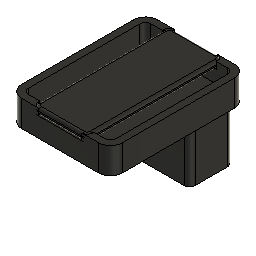
IMUmount (Autodesk Fusion 360 design; units mm, degrees)
Autodesk Fusion 360 part; units mm, degrees
sketch "Sketch1" plane through (0, 0, -6.0198) normal (0, 0, 1) x (-1, 0, 0)
  line L0 (-4.0409, -57.15) -> (2.9359, -57.15)
  line L1 (2.9359, -57.15) -> (3.9347, -56.1512)
  line L2 (3.9347, -56.1512) -> (3.9347, 6.35)
  line L3 (3.9347, 6.35) -> (-16.6393, 6.35)
  line L4 (-16.6393, 6.35) -> (-16.6393, -56.1512)
  line L5 (-16.6393, -56.1512) -> (-15.6405, -57.15)
  line L6 (-15.6405, -57.15) -> (-8.6637, -57.15)
  line L7 (-8.6637, -57.15) -> (-8.6637, -55.3466)
  arc A0 (-8.1557, -54.8386) -> (-8.6637, -55.3466) centre (-8.1557, -55.3466) ccw
  line L8 (-8.1557, -54.8386) -> (-4.5489, -54.8386)
  arc A1 (-4.0409, -55.3466) -> (-4.5489, -54.8386) centre (-4.5489, -55.3466) ccw
  line L9 (-4.0409, -55.3466) -> (-4.0409, -57.15)
  arc A2 (-8.1557, -42.1386) -> (-8.6637, -42.6466) centre (-8.1557, -42.6466) ccw
  line L10 (-8.1557, -42.1386) -> (-4.5489, -42.1386)
  arc A3 (-4.0409, -42.6466) -> (-4.5489, -42.1386) centre (-4.5489, -42.6466) ccw
  line L11 (-4.0409, -42.6466) -> (-4.0409, -46.2534)
  arc A4 (-4.5489, -46.7614) -> (-4.0409, -46.2534) centre (-4.5489, -46.2534) ccw
  line L12 (-4.5489, -46.7614) -> (-8.1557, -46.7614)
  arc A5 (-8.6637, -46.2534) -> (-8.1557, -46.7614) centre (-8.1557, -46.2534) ccw
  line L13 (-8.6637, -46.2534) -> (-8.6637, -42.6466)
  arc A6 (-8.1557, -29.4386) -> (-8.6637, -29.9466) centre (-8.1557, -29.9466) ccw
  line L14 (-8.1557, -29.4386) -> (-4.5489, -29.4386)
  arc A7 (-4.0409, -29.9466) -> (-4.5489, -29.4386) centre (-4.5489, -29.9466) ccw
  line L15 (-4.0409, -29.9466) -> (-4.0409, -33.5534)
  arc A8 (-4.5489, -34.0614) -> (-4.0409, -33.5534) centre (-4.5489, -33.5534) ccw
  line L16 (-4.5489, -34.0614) -> (-8.1557, -34.0614)
  arc A9 (-8.6637, -33.5534) -> (-8.1557, -34.0614) centre (-8.1557, -33.5534) ccw
  line L17 (-8.6637, -33.5534) -> (-8.6637, -29.9466)
  arc A10 (1.8011, -53.1114) -> (2.3091, -52.6034) centre (1.8011, -52.6034) ccw
  line L18 (1.8011, -53.1114) -> (-1.8057, -53.1114)
  arc A11 (-2.3137, -52.6034) -> (-1.8057, -53.1114) centre (-1.8057, -52.6034) ccw
  line L19 (-2.3137, -52.6034) -> (-2.3137, -48.9966)
  arc A12 (-1.8057, -48.4886) -> (-2.3137, -48.9966) centre (-1.8057, -48.9966) ccw
  line L20 (-1.8057, -48.4886) -> (1.8011, -48.4886)
  arc A13 (2.3091, -48.9966) -> (1.8011, -48.4886) centre (1.8011, -48.9966) ccw
  line L21 (2.3091, -48.9966) -> (2.3091, -52.6034)
  arc A14 (1.8011, -40.4114) -> (2.3091, -39.9034) centre (1.8011, -39.9034) ccw
  line L22 (1.8011, -40.4114) -> (-1.8057, -40.4114)
  arc A15 (-2.3137, -39.9034) -> (-1.8057, -40.4114) centre (-1.8057, -39.9034) ccw
  line L23 (-2.3137, -39.9034) -> (-2.3137, -36.2966)
  arc A16 (-1.8057, -35.7886) -> (-2.3137, -36.2966) centre (-1.8057, -36.2966) ccw
  line L24 (-1.8057, -35.7886) -> (1.8011, -35.7886)
  arc A17 (2.3091, -36.2966) -> (1.8011, -35.7886) centre (1.8011, -36.2966) ccw
  line L25 (2.3091, -36.2966) -> (2.3091, -39.9034)
  arc A18 (1.8011, -27.7114) -> (2.3091, -27.2034) centre (1.8011, -27.2034) ccw
  line L26 (1.8011, -27.7114) -> (-1.8057, -27.7114)
  arc A19 (-2.3137, -27.2034) -> (-1.8057, -27.7114) centre (-1.8057, -27.2034) ccw
  line L27 (-2.3137, -27.2034) -> (-2.3137, -23.5966)
  arc A20 (-1.8057, -23.0886) -> (-2.3137, -23.5966) centre (-1.8057, -23.5966) ccw
  line L28 (-1.8057, -23.0886) -> (1.8011, -23.0886)
  arc A21 (2.3091, -23.5966) -> (1.8011, -23.0886) centre (1.8011, -23.5966) ccw
  line L29 (2.3091, -23.5966) -> (2.3091, -27.2034)
  arc A22 (1.8011, -15.0114) -> (2.3091, -14.5034) centre (1.8011, -14.5034) ccw
  line L30 (1.8011, -15.0114) -> (-1.8057, -15.0114)
  arc A23 (-2.3137, -14.5034) -> (-1.8057, -15.0114) centre (-1.8057, -14.5034) ccw
  line L31 (-2.3137, -14.5034) -> (-2.3137, -10.8966)
  arc A24 (-1.8057, -10.3886) -> (-2.3137, -10.8966) centre (-1.8057, -10.8966) ccw
  line L32 (-1.8057, -10.3886) -> (1.8011, -10.3886)
  arc A25 (2.3091, -10.8966) -> (1.8011, -10.3886) centre (1.8011, -10.8966) ccw
  line L33 (2.3091, -10.8966) -> (2.3091, -14.5034)
  arc A26 (1.8011, -2.3114) -> (2.3091, -1.8034) centre (1.8011, -1.8034) ccw
  line L34 (1.8011, -2.3114) -> (-1.8057, -2.3114)
  arc A27 (-2.3137, -1.8034) -> (-1.8057, -2.3114) centre (-1.8057, -1.8034) ccw
  line L35 (-2.3137, -1.8034) -> (-2.3137, 1.8034)
  arc A28 (-1.8057, 2.3114) -> (-2.3137, 1.8034) centre (-1.8057, 1.8034) ccw
  line L36 (-1.8057, 2.3114) -> (1.8011, 2.3114)
  arc A29 (2.3091, 1.8034) -> (1.8011, 2.3114) centre (1.8011, 1.8034) ccw
  line L37 (2.3091, 1.8034) -> (2.3091, -1.8034)
  arc A30 (-10.8989, -53.1114) -> (-10.3909, -52.6034) centre (-10.8989, -52.6034) ccw
  line L38 (-10.8989, -53.1114) -> (-14.5057, -53.1114)
  arc A31 (-15.0137, -52.6034) -> (-14.5057, -53.1114) centre (-14.5057, -52.6034) ccw
  line L39 (-15.0137, -52.6034) -> (-15.0137, -48.9966)
  arc A32 (-14.5057, -48.4886) -> (-15.0137, -48.9966) centre (-14.5057, -48.9966) ccw
  line L40 (-14.5057, -48.4886) -> (-10.8989, -48.4886)
  arc A33 (-10.3909, -48.9966) -> (-10.8989, -48.4886) centre (-10.8989, -48.9966) ccw
  line L41 (-10.3909, -48.9966) -> (-10.3909, -52.6034)
  arc A34 (-10.8989, -40.4114) -> (-10.3909, -39.9034) centre (-10.8989, -39.9034) ccw
  line L42 (-10.8989, -40.4114) -> (-14.5057, -40.4114)
  arc A35 (-15.0137, -39.9034) -> (-14.5057, -40.4114) centre (-14.5057, -39.9034) ccw
  line L43 (-15.0137, -39.9034) -> (-15.0137, -36.2966)
  arc A36 (-14.5057, -35.7886) -> (-15.0137, -36.2966) centre (-14.5057, -36.2966) ccw
  line L44 (-14.5057, -35.7886) -> (-10.8989, -35.7886)
  arc A37 (-10.3909, -36.2966) -> (-10.8989, -35.7886) centre (-10.8989, -36.2966) ccw
  line L45 (-10.3909, -36.2966) -> (-10.3909, -39.9034)
  arc A38 (-10.8989, -27.7114) -> (-10.3909, -27.2034) centre (-10.8989, -27.2034) ccw
  line L46 (-10.8989, -27.7114) -> (-14.5057, -27.7114)
  arc A39 (-15.0137, -27.2034) -> (-14.5057, -27.7114) centre (-14.5057, -27.2034) ccw
  line L47 (-15.0137, -27.2034) -> (-15.0137, -23.5966)
  arc A40 (-14.5057, -23.0886) -> (-15.0137, -23.5966) centre (-14.5057, -23.5966) ccw
  line L48 (-14.5057, -23.0886) -> (-10.8989, -23.0886)
  arc A41 (-10.3909, -23.5966) -> (-10.8989, -23.0886) centre (-10.8989, -23.5966) ccw
  line L49 (-10.3909, -23.5966) -> (-10.3909, -27.2034)
  arc A42 (-10.8989, -15.0114) -> (-10.3909, -14.5034) centre (-10.8989, -14.5034) ccw
  line L50 (-10.8989, -15.0114) -> (-14.5057, -15.0114)
  arc A43 (-15.0137, -14.5034) -> (-14.5057, -15.0114) centre (-14.5057, -14.5034) ccw
  line L51 (-15.0137, -14.5034) -> (-15.0137, -10.8966)
  arc A44 (-14.5057, -10.3886) -> (-15.0137, -10.8966) centre (-14.5057, -10.8966) ccw
  line L52 (-14.5057, -10.3886) -> (-10.8989, -10.3886)
  arc A45 (-10.3909, -10.8966) -> (-10.8989, -10.3886) centre (-10.8989, -10.8966) ccw
  line L53 (-10.3909, -10.8966) -> (-10.3909, -14.5034)
  arc A46 (-10.8989, -2.3114) -> (-10.3909, -1.8034) centre (-10.8989, -1.8034) ccw
  line L54 (-10.8989, -2.3114) -> (-14.5057, -2.3114)
  arc A47 (-15.0137, -1.8034) -> (-14.5057, -2.3114) centre (-14.5057, -1.8034) ccw
  line L55 (-15.0137, -1.8034) -> (-15.0137, 1.8034)
  arc A48 (-14.5057, 2.3114) -> (-15.0137, 1.8034) centre (-14.5057, 1.8034) ccw
  line L56 (-14.5057, 2.3114) -> (-10.8989, 2.3114)
  arc A49 (-10.3909, 1.8034) -> (-10.8989, 2.3114) centre (-10.8989, 1.8034) ccw
  line L57 (-10.3909, 1.8034) -> (-10.3909, -1.8034)
  arc A50 (-8.6637, -8.1534) -> (-8.1557, -8.6614) centre (-8.1557, -8.1534) ccw
  line L58 (-8.6637, -8.1534) -> (-8.6637, -4.5466)
  arc A51 (-8.1557, -4.0386) -> (-8.6637, -4.5466) centre (-8.1557, -4.5466) ccw
  line L59 (-8.1557, -4.0386) -> (-4.5489, -4.0386)
  arc A52 (-4.0409, -4.5466) -> (-4.5489, -4.0386) centre (-4.5489, -4.5466) ccw
  line L60 (-4.0409, -4.5466) -> (-4.0409, -8.1534)
  arc A53 (-4.5489, -8.6614) -> (-4.0409, -8.1534) centre (-4.5489, -8.1534) ccw
  line L61 (-4.5489, -8.6614) -> (-8.1557, -8.6614)
  arc A54 (-8.1557, -16.7386) -> (-8.6637, -17.2466) centre (-8.1557, -17.2466) ccw
  line L62 (-8.1557, -16.7386) -> (-4.5489, -16.7386)
  arc A55 (-4.0409, -17.2466) -> (-4.5489, -16.7386) centre (-4.5489, -17.2466) ccw
  line L63 (-4.0409, -17.2466) -> (-4.0409, -20.8534)
  arc A56 (-4.5489, -21.3614) -> (-4.0409, -20.8534) centre (-4.5489, -20.8534) ccw
  line L64 (-4.5489, -21.3614) -> (-8.1557, -21.3614)
  arc A57 (-8.6637, -20.8534) -> (-8.1557, -21.3614) centre (-8.1557, -20.8534) ccw
  line L65 (-8.6637, -20.8534) -> (-8.6637, -17.2466)
  line L66 (2.6647, -56.1512) -> (-15.3693, -56.1512)
  line L67 (-16.6393, -54.8812) -> (-16.6393, -47.2612)
  line L68 (-15.3693, -45.9912) -> (2.6647, -45.9912)
  line L69 (3.9347, -47.2612) -> (3.9347, -54.8812)
  arc A58 (2.6647, -56.1512) -> (3.9347, -54.8812) centre (2.6647, -54.8812) ccw
  arc A59 (3.9347, -47.2612) -> (2.6647, -45.9912) centre (2.6647, -47.2612) ccw
  arc A60 (-15.3693, -45.9912) -> (-16.6393, -47.2612) centre (-15.3693, -47.2612) ccw
  arc A61 (-16.6393, -54.8812) -> (-15.3693, -56.1512) centre (-15.3693, -54.8812) ccw
  point P0 (-16.6393, -56.1512)
  point P1 (-16.6393, -45.9912)
  dimension "d1" = 10.16
  dimension "d2" = 1.27
  constraint coincident P0 L4.end
  constraint coincident L4 P1
  constraint perpendicular L2 L68
  constraint tangent L66 A58
  constraint tangent L69 A58
  constraint tangent L68 A59
  constraint tangent L69 A59
  constraint equal A58 A59
  constraint coincident P1 L67
  constraint coincident P1 L68
  constraint tangent L67 A60
  constraint tangent L68 A60
  constraint equal A58 A60
  constraint coincident P0 L66
  constraint coincident P0 L67
  constraint tangent L66 A61
  constraint tangent L67 A61
  constraint equal A58 A61
  measures "d1" distance of P0 P1
  measures "d2" radius of A58
extrude "Extrude1" add sketch "Sketch1" along normal blind 12.7 contours L7 A0 L8 A1 L9 L66 | L2 L4 L7 A0 L8 A1 L9 L11 A4 L12 A5 L13 L66 L67 L68 L69 A58 A59 A60 A61 | L11 A4 L12 A5 L13 L68 | A10 L18 A11 L19 A12 L20 A13 L21 | A30 L38 A31 L39 A32 L40 A33 L41 makes body 1
sketch "Sketch2" plane through (0, 0, 6.6802) normal (0, 0, 1) x (-1, 0, 0)
  arc A0 (-15.3693, -45.9912) -> (-16.6393, -47.2612) centre (-15.3693, -47.2612) ccw
  line L0 (-16.6393, -47.2612) -> (-16.6393, -54.8812)
  arc A1 (-16.6393, -54.8812) -> (-15.3693, -56.1512) centre (-15.3693, -54.8812) ccw
  line L1 (-15.3693, -56.1512) -> (2.6647, -56.1512)
  arc A2 (2.6647, -56.1512) -> (3.9347, -54.8812) centre (2.6647, -54.8812) ccw
  line L2 (3.9347, -54.8812) -> (3.9347, -47.2612)
  arc A3 (3.9347, -47.2612) -> (2.6647, -45.9912) centre (2.6647, -47.2612) ccw
  line L3 (2.6647, -45.9912) -> (-15.3693, -45.9912)
  line L4 (3.9347, -54.8812) -> (3.9347, -28.6512)
  line L5 (2.6647, -27.3812) -> (-15.3693, -27.3812)
  line L6 (-16.6393, -28.6512) -> (-16.6393, -54.8812)
  arc A4 (3.9347, -28.6512) -> (2.6647, -27.3812) centre (2.6647, -28.6512) ccw
  arc A5 (-15.3693, -27.3812) -> (-16.6393, -28.6512) centre (-15.3693, -28.6512) ccw
  line L7 (2.6653, -56.1907) -> (-15.3699, -56.1907)
  arc A6 (2.6653, -56.1907) -> (3.9347, -54.8812) centre (2.6653, -54.9207) ccw
  arc A7 (-16.6393, -54.8812) -> (-15.3699, -56.1907) centre (-15.3699, -54.9207) ccw
  arc A8 (-18.2268, -54.8615) -> (-15.3699, -57.7782) centre (-15.3699, -54.9207) ccw
  line L8 (2.6653, -57.7782) -> (-15.3699, -57.7782)
  arc A9 (2.6653, -57.7782) -> (5.5222, -54.8615) centre (2.6653, -54.9207) ccw
  line L9 (5.5222, -54.8615) -> (5.5222, -28.6512)
  arc A10 (5.5222, -28.6512) -> (2.6647, -25.7937) centre (2.6647, -28.6512) ccw
  line L10 (2.6647, -25.7937) -> (-15.3693, -25.7937)
  arc A11 (-15.3693, -25.7937) -> (-18.2268, -28.6512) centre (-15.3693, -28.6512) ccw
  line L11 (-18.2268, -28.6512) -> (-18.2268, -54.8615)
  point P0 (3.9347, -27.3812)
  dimension "d5" = 27.5
  dimension "d6" = 1.27
  dimension "d7" = 1.27
  dimension "d8" = -1.5875
  constraint coincident A2.end L2.start
  constraint tangent A2 L4
  constraint perpendicular L0 L5
  constraint coincident L0.end A1.start
  constraint tangent A1 L6
  constraint coincident P0 L4
  constraint coincident P0 L5
  constraint tangent L4 A4
  constraint tangent L5 A4
  constraint tangent L5 A5
  constraint tangent L6 A5
  constraint equal A4 A5
  constraint perpendicular L0 L7
  constraint tangent L7 A6
  constraint tangent L7 A7
  constraint equal A6 A7
  measures "d5" distance of A2.end P0
  measures "d6" radius of A4
  measures "d7" radius of A6
extrude "Extrude2" add sketch "Sketch2" along normal blind 4.572 separate body makes body 2
sketch "Sketch3" plane through (0, 0, 6.6802) normal (0, 0, -1) x (1, 0, 0)
  arc A0 (-3.9347, -54.8812) -> (-2.6653, -56.1907) centre (-2.6653, -54.9207) ccw
  line L0 (-3.9347, -54.8812) -> (-3.9347, -28.6512)
  arc A1 (-2.6647, -27.3812) -> (-3.9347, -28.6512) centre (-2.6647, -28.6512) ccw
  line L1 (-2.6647, -27.3812) -> (15.3693, -27.3812)
  arc A2 (16.6393, -28.6512) -> (15.3693, -27.3812) centre (15.3693, -28.6512) ccw
  line L2 (16.6393, -28.6512) -> (16.6393, -54.8812)
  arc A3 (15.3699, -56.1907) -> (16.6393, -54.8812) centre (15.3699, -54.9207) ccw
  line L3 (15.3699, -56.1907) -> (-2.6653, -56.1907)
  arc A4 (-5.5222, -54.8615) -> (-2.6653, -57.7782) centre (-2.6653, -54.9207) ccw
  line L4 (-2.6653, -57.7782) -> (15.3699, -57.7782)
  arc A5 (15.3699, -57.7782) -> (18.2268, -54.8615) centre (15.3699, -54.9207) ccw
  line L5 (18.2268, -54.8615) -> (18.2268, -28.6512)
  arc A6 (18.2268, -28.6512) -> (15.3693, -25.7937) centre (15.3693, -28.6512) ccw
  line L6 (15.3693, -25.7937) -> (-2.6647, -25.7937)
  arc A7 (-2.6647, -25.7937) -> (-5.5222, -28.6512) centre (-2.6647, -28.6512) ccw
  line L7 (-5.5222, -28.6512) -> (-5.5222, -54.8615)
extrude "Extrude3" add sketch "Sketch3" against normal blind 1.5875 contours A0 L0 A1 L1 A2 L2 A3 L3 bodies 1 2
extrude "Extrude9" add 1 faces at (-4.4638, 46.1313, 11.2522) along direction (0, 0, 1) blind 1.5875 on bodies 1 bodies 1
sketch "Sketch11" plane through (0, 0, 12.8397) normal (0, 0, 1) x (-1, 0, 0)
  line L0 (3.9347, -28.6512) -> (3.9347, -54.8812)
  arc A0 (2.6653, -56.1907) -> (3.9347, -54.8812) centre (2.6653, -54.9207) ccw
  line L1 (2.6653, -56.1907) -> (-15.3699, -56.1907)
  arc A1 (-16.6393, -54.8812) -> (-15.3699, -56.1907) centre (-15.3699, -54.9207) ccw
  line L2 (-16.6393, -54.8812) -> (-16.6393, -28.6512)
  arc A2 (-15.3693, -27.3812) -> (-16.6393, -28.6512) centre (-15.3693, -28.6512) ccw
  line L3 (-15.3693, -27.3812) -> (2.6647, -27.3812)
  arc A3 (3.9347, -28.6512) -> (2.6647, -27.3812) centre (2.6647, -28.6512) ccw
  arc A4 (2.6653, -57.7782) -> (5.5222, -54.8615) centre (2.6653, -54.9207) ccw
  line L4 (5.5222, -54.8615) -> (5.5222, -28.6512)
  arc A5 (5.5222, -28.6512) -> (2.6647, -25.7937) centre (2.6647, -28.6512) ccw
  line L5 (2.6647, -25.7937) -> (-15.3693, -25.7937)
  arc A6 (-15.3693, -25.7937) -> (-18.2268, -28.6512) centre (-15.3693, -28.6512) ccw
  line L6 (-18.2268, -28.6512) -> (-18.2268, -54.8615)
  arc A7 (-18.2268, -54.8615) -> (-15.3699, -57.7782) centre (-15.3699, -54.9207) ccw
  line L7 (-15.3699, -57.7782) -> (2.6653, -57.7782)
  line L8 (-6.3523, -57.7782) -> (-1.2723, -57.7782)
  line L9 (-6.3523, -57.7782) -> (-11.4323, -57.7782)
  line L10 (-12.7023, -56.5082) -> (-12.7023, -27.0637)
  line L11 (-11.4323, -25.7937) -> (-1.2723, -25.7937)
  line L12 (-0.0023, -27.0637) -> (-0.0023, -56.5082)
  arc A8 (-11.4323, -25.7937) -> (-12.7023, -27.0637) centre (-11.4323, -27.0637) ccw
  arc A9 (-0.0023, -27.0637) -> (-1.2723, -25.7937) centre (-1.2723, -27.0637) ccw
  arc A10 (-1.2723, -57.7782) -> (-0.0023, -56.5082) centre (-1.2723, -56.5082) ccw
  arc A11 (-12.7023, -56.5082) -> (-11.4323, -57.7782) centre (-11.4323, -56.5082) ccw
  point P0 (-0.0023, -57.7782)
  point P1 (-12.7023, -57.7782)
  point P2 (-12.7023, -25.7937)
  point P3 (-0.0023, -25.7937)
  dimension "d46" = 6.35
  dimension "d47" = 6.35
  dimension "d48" = 12.7
  dimension "d49" = 1.27
  constraint midpoint L7 L8.start
  constraint coincident L7 P0
  constraint coincident L7 P1
  constraint coincident L5 P2
  constraint perpendicular L5 L10
  constraint coincident L5 P3
  constraint coincident P2 L10
  constraint coincident P2 L11
  constraint tangent L10 A8
  constraint tangent L11 A8
  constraint coincident P3 L11
  constraint coincident P3 L12
  constraint tangent L11 A9
  constraint tangent L12 A9
  constraint equal A8 A9
  constraint coincident P0 L8
  constraint coincident P0 L12
  constraint tangent L8 A10
  constraint tangent L12 A10
  constraint equal A8 A10
  constraint coincident P1 L9
  constraint coincident P1 L10
  constraint tangent L9 A11
  constraint tangent L10 A11
  constraint equal A8 A11
  measures "d46" distance of L8.start P0
  measures "d47" distance of L8.start P1
  measures "d48" distance of P2 P3
  measures "d49" radius of A8
extrude "Extrude10" cut sketch "Sketch11" against normal blind 1.5875 contours L3 L5 L10 L11 L12 A8 A9 | L1 L7 L8 L9 L10 L12 A10 A11 bodies 1
extrude "Extrude11" add sketch "Sketch11" along normal blind 1.5875 separate body contours L1 L3 L10 L12 | L3 L5 L10 L11 L12 A8 A9 | L1 L7 L8 L9 L10 L12 A10 A11 makes body 3
move_body "Move1" bodies 3 to x (1, 0, 0) y (0, 1, 0) z (0, 0, 1) at (24.4142, 0, 0)
fillet "Fillet3" radius 0.635 16 edges at (30.7666, 57.7782, 14.4272) (24.7885, 57.4062, 14.4272) (24.4166, 41.7859, 14.4272) (24.7885, 26.1657, 14.4272) (30.7666, 25.7937, 14.4272) (36.7446, 26.1657, 14.4272) (37.1166, 41.7859, 14.4272) (36.7446, 57.4062, 14.4272) (36.7446, 26.1657, 12.8397) (30.7666, 25.7937, 12.8397) (24.7885, 26.1657, 12.8397) (24.4166, 41.7859, 12.8397) (24.7885, 57.4062, 12.8397) (30.7666, 57.7782, 12.8397) (36.7446, 57.4062, 12.8397) (37.1166, 41.7859, 12.8397) on bodies 3
hole "Hole3" at (12.7, 50.8, -6.0198) direction (0, 0, 1) diameter 3.429 depth 9.525 tip angle 180 bodies 1
thread "Thread3" "ANSI Unified Screw Threads 0.164(#8) 8-32 UNC 8-32 UNC 2B" major diameter 4.1656 minor diameter 3.4163 pitch 0.7937 angle 60 modelled right hand crest width 0.2341 on face at (12.8707, 52.506, -2.8448) crest through (10.9919, 50.8, -5.8214) on bodies 1
hole "Hole4" at (0, 50.8, -6.0198) direction (0, 0, 1) diameter 3.429 depth 9.525 tip angle 180 bodies 1
thread "Thread4" "ANSI Unified Screw Threads 0.164(#8) 8-32 UNC 8-32 UNC 2B" major diameter 4.1656 minor diameter 3.4163 pitch 0.7937 angle 60 modelled right hand crest width 0.2341 on face at (0.1707, 52.506, -2.8448) crest through (-1.7081, 50.8, -5.8214) on bodies 1
move_body "Move2" bodies 3 to x (1, 0, 0) y (0, 1, 0) z (0, 0, 1) at (-24.3869, 0, -1.5775)
equation "d8 = ( -1 / 16 ) * 1 in"
equation "d11 = ( -1 / 16 ) * 1 in"
equation "d44 = ( 1 / 16 ) * 1 in"
equation "d50 = ( -1 / 16 ) * 1 in"
equation "d52 = ( 1 / 16 ) * 1 in"
named bodies: "IMUmount", "IMUcover"
